Autodesk Inventor part; units mm, degrees
(part 2 of 3)
sketch "Эскиз19" plane through (0, 0, 0) normal (0, 1, 0) x (-1, 0, 0)
  arc A0 (-28.0199, 71.0163) -> (28.0199, 71.0163) centre (0, 104.941) ccw construction
  arc A1 (-23.7825, 76.5969) -> (23.7825, 76.5969) centre (0, 104.941) ccw construction
  line L0 (0, 0) -> (0, 95.3237) construction
  circle A2 centre (0, 56.2966) radius 3.05 construction
  circle A3 centre (0, 56.2966) radius 1.55 construction
  arc A4 (-0.6161, 51.9466) -> (0.6161, 51.9466) centre (0, 53.8493) ccw construction
  arc A5 (-0.6161, 59.3045) -> (0.6161, 59.3045) centre (0, 61.2072) ccw construction
  line L1 (0, 59.2072) -> (0, 51.8493) construction
  arc A6 (0.6251, 60.6437) -> (-0.6251, 60.6437) centre (0, 58.7439) ccw construction
  line L2 (0, 60.7439) -> (0, 51.8493) construction
  line L3 (0, 56.2966) -> (1.525, 58.938) construction
  line L4 (0, 56.2966) -> (-1.525, 58.938) construction
  line L5 (0, 56.2966) -> (-3.05, 56.2966) construction
  line L6 (0, 56.2966) -> (-1.525, 53.6552) construction
  line L7 (0, 56.2966) -> (1.525, 53.6552) construction
  line L8 (0, 56.2966) -> (3.05, 56.2966) construction
  line L9 (1.525, 58.938) -> (3.05, 56.2966) construction
  line L10 (1.525, 53.6552) -> (3.05, 56.2966) construction
  line L11 (1.525, 53.6552) -> (-1.525, 53.6552) construction
  line L12 (-1.525, 53.6552) -> (-3.05, 56.2966) construction
  line L13 (-3.05, 56.2966) -> (-1.525, 58.938) construction
  line L14 (-1.525, 58.938) -> (1.525, 58.938) construction
  arc A7 (0, 51.2466) -> (4.3734, 53.7716) centre (0, 56.2966) ccw construction
  arc A8 (-28.0199, 71.0163) -> (28.0199, 71.0163) centre (0, 104.941) ccw construction
  line L15 (9.0567, 61.8832) -> (4.3734, 53.7716) construction
  line L16 (-9.0567, 61.8832) -> (-4.3734, 53.7716) construction
  arc A9 (-4.3734, 53.7716) -> (0, 51.2466) centre (0, 56.2966) ccw construction
  arc A10 (4.3734, 53.7716) -> (-4.3734, 53.7716) centre (0, 56.2966) ccw construction
  arc A11 (-9.0567, 61.8832) -> (9.0567, 61.8832) centre (0, 104.941) ccw construction
  arc A12 (-9.0567, 61.8832) -> (9.0567, 61.8832) centre (0, 104.941) ccw construction
  line L17 (0, 57.8466) -> (0, 54.7466) construction
  circle A13 centre (-20.558, 60.8542) radius 3.25 construction
  circle A14 centre (-20.558, 60.8542) radius 1.7
  line L18 (-19.3274, 63.4932) -> (-22.4408, 56.8165) construction
  line L19 (-18.6752, 64.8919) -> (-22.4408, 56.8165) construction
  line L20 (-20.558, 60.8542) -> (-17.8958, 62.7183) construction
  line L21 (-20.558, 60.8542) -> (-20.8413, 64.0918) construction
  line L22 (-20.558, 60.8542) -> (-23.5035, 62.2277) construction
  line L23 (-20.558, 60.8542) -> (-23.2203, 58.9901) construction
  line L24 (-20.558, 60.8542) -> (-20.2748, 57.6166) construction
  line L25 (-20.558, 60.8542) -> (-17.6125, 59.4807) construction
  line L26 (-17.8958, 62.7183) -> (-17.6125, 59.4807)
  line L27 (-20.2748, 57.6166) -> (-17.6125, 59.4807)
  line L28 (-20.2748, 57.6166) -> (-23.2203, 58.9901)
  line L29 (-23.2203, 58.9901) -> (-23.5035, 62.2277)
  line L30 (-23.5035, 62.2277) -> (-20.8413, 64.0918)
  line L31 (-20.8413, 64.0918) -> (-17.8958, 62.7183)
  arc A15 (-22.7768, 56.0961) -> (-17.5013, 56.5858) centre (-20.558, 60.8542) ccw
  line L32 (-9.8579, 62.0595) -> (-17.5013, 56.5858)
  line L33 (-26.4019, 69.7424) -> (-25.788, 60.3966)
  arc A16 (-25.788, 60.3966) -> (-22.7768, 56.0961) centre (-20.558, 60.8542) ccw
  arc A17 (-17.5013, 56.5858) -> (-25.788, 60.3966) centre (-20.558, 60.8542) ccw construction
  arc A18 (-26.3973, 69.6727) -> (-9.931, 62.0072) centre (0, 104.8583) ccw construction
  arc A19 (-26.3973, 69.6727) -> (-9.931, 62.0072) centre (0, 104.8583) ccw construction
  line L34 (-19.8396, 62.3949) -> (-21.2765, 59.3135) construction
  arc A20 (-26.4052, 69.7449) -> (-9.8579, 62.0595) centre (0, 104.941) ccw
  line L35 (20.558, 60.8542) -> (20.8413, 64.0918) construction
  line L36 (20.8413, 64.0918) -> (17.8958, 62.7183)
  line L37 (23.5035, 62.2277) -> (20.8413, 64.0918)
  line L38 (20.558, 60.8542) -> (23.5035, 62.2277) construction
  circle A21 centre (20.558, 60.8542) radius 1.7
  line L39 (20.558, 60.8542) -> (23.2203, 58.9901) construction
  line L40 (20.2748, 57.6166) -> (23.2203, 58.9901)
  line L41 (19.3274, 63.4932) -> (22.4408, 56.8165) construction
  circle A22 centre (20.558, 60.8542) radius 3.25 construction
  line L42 (18.6752, 64.8919) -> (22.4408, 56.8165) construction
  arc A23 (25.788, 60.3966) -> (17.5013, 56.5858) centre (20.558, 60.8542) ccw construction
  arc A24 (22.7768, 56.0961) -> (25.788, 60.3966) centre (20.558, 60.8542) ccw
  line L43 (20.558, 60.8542) -> (17.8958, 62.7183) construction
  line L44 (26.4019, 69.7424) -> (25.788, 60.3966)
  line L45 (23.2203, 58.9901) -> (23.5035, 62.2277)
  arc A25 (9.931, 62.0072) -> (26.3973, 69.6727) centre (0, 104.8583) ccw construction
  arc A26 (9.931, 62.0072) -> (26.3973, 69.6727) centre (0, 104.8583) ccw construction
  line L46 (19.8396, 62.3949) -> (21.2765, 59.3135) construction
  line L47 (20.558, 60.8542) -> (20.2748, 57.6166) construction
  line L48 (20.558, 60.8542) -> (17.6125, 59.4807) construction
  line L49 (17.8958, 62.7183) -> (17.6125, 59.4807)
  line L50 (20.2748, 57.6166) -> (17.6125, 59.4807)
  line L51 (9.8579, 62.0595) -> (17.5013, 56.5858)
  arc A27 (17.5013, 56.5858) -> (22.7768, 56.0961) centre (20.558, 60.8542) ccw
  arc A28 (9.8579, 62.0595) -> (26.4052, 69.7449) centre (0, 104.941) ccw
  point P0 (0, 55.5283)
  point P1 (-20.8841, 60.1549)
  point P2 (-9.9889, 62.0899)
  point P3 (20.8841, 60.1549)
  point P4 (9.9889, 62.0899)
  point P5 (9.9889, 62.0899)
  point P6 (-9.9889, 62.0899)
  dimension "d154" = 6.1
  dimension "d155" = 3.1
  dimension "d166" = 360
  dimension "d168" = 2
  dimension "d169" = 30
  dimension "d178" = 6.5
  dimension "d179" = 3.4
  dimension "d180" = 360
  dimension "d181" = 2
  constraints: 102 end point, 56 point on circle, 32 symmetric about line, 23 centre point, 15 point on line, 12 coincident, 6 parallel, 4 midpoint, 4 tangent, 2 perpendicular, 1 collinear, 1 vertical, 47 other
  measures "d154" diameter of A2
  measures "d155" diameter of A3
  measures "d168" radial gap between concentric circles of A7 A2
  measures "d169" angle of L0 L15
  measures "d178" diameter of A13
  measures "d179" diameter of A14
  measures "d181" radial gap between concentric circles of A15 A13
extrude "Выдавливание15" add sketch "Эскиз19" along normal blind 3 contours L26 L27 L28 L29 L30 L31 | L37 L45 L40 L50 L49 L36
extrude "Выдавливание16" add sketch "Эскиз19" along normal blind 10 contours A16 L33 A20 L32 A15 | A27 L51 A28 L44 A24
ref_plane "РабПлоскость7" through (21.7475, 10, 58.3033) normal (0.9063078, 0, 0.4226183) x (0, 1, 0)
sketch "Эскиз22" plane through (21.7475, 10, 58.3033) normal (0.9063078, 0, 0.4226183) x (0, 1, 0)
  line L0 (-10, 51.459) -> (30.2664, 51.459)
  line L1 (-10, -2.4354) -> (-10, 0.1896) construction
  line L2 (-10, -2.4354) -> (-5, -2.4354) construction
  line L3 (-10, -2.4354) -> (0, -2.4354) construction
  line L4 (-5, -2.4354) -> (9.5622, -2.4354) construction
  line L5 (0, 7.459) -> (0, 8.4003) construction
  line L6 (-5, -2.4354) -> (5, -2.4354)
  line L7 (-5, -2.4354) -> (0, 7.459)
  line L8 (0, 7.459) -> (20, 7.459) construction
  line L9 (0, 7.459) -> (5, 7.459)
  line L10 (5, 7.459) -> (5, -2.4354)
  point P0 (-10, -43.6499)
  dimension "d190" = 5
  dimension "d191" = 10
  constraints: 14 end point, 3 point on line, 1 horizontal, 1 midpoint, 1 perpendicular
  measures "d190" distance of L1.start L2.end
  measures "d191" distance of L2.end L6.end
ref_plane "РабПлоскость9" through (-21.7475, 10, 58.3033) normal (-0.9063078, 0, 0.4226183) x (0, -1, 0)
sketch "Эскиз25" plane through (-21.7475, 10, 58.3033) normal (-0.9063078, 0, 0.4226183) x (0, -1, 0)
  line L0 (0, 7.459) -> (-20, 7.459) construction
  line L1 (10, -2.4354) -> (0, -2.4354) construction
  line L2 (10, 0.2379) -> (10, -2.4354) construction
  line L3 (10, -2.4354) -> (5, -2.4354) construction
  line L4 (0, 8.4291) -> (0, 7.459) projected
  line L5 (5, -2.4354) -> (0, 7.459)
  line L6 (0, 7.459) -> (-5, 7.459)
  line L7 (10, 51.459) -> (0, 51.459)
  line L8 (10, 0.2379) -> (10, 0.1896) projected
  line L9 (10, 0.1896) -> (0, 0.1896) projected
  line L10 (0, 0.2379) -> (0, 0.1896) projected
  line L11 (10, 0.2379) -> (0, 0.2379) projected
  line L12 (10, -2.4354) -> (0, -2.4354) projected
  line L13 (5, -2.4354) -> (-4.0389, -6.1705)
  line L14 (-4.0389, -6.1705) -> (-5, 7.459)
  point P0 (10, -43.6499)
  dimension "d192" = 5
  dimension "d193" = 5
  dimension "d194" = 10
  constraints: 12 end point, 1 horizontal, 1 midpoint, 1 point on line
  measures "d192" distance of L1.start L3.end
  measures "d193" distance of L0.start L6.end
  measures "d194" distance of L7.start L7.end
ref_plane "РабПлоскость10" through (0, 0, 69.1191) normal (1, 0, 0) x (0, -1, 0)
sketch "Эскиз26" plane through (0, 0, 69.1191) normal (1, 0, 0) x (0, -1, 0)
  line L0 (0, 8.178) -> (-30, 8.178) projected
  line L1 (0, 17.8725) -> (0, 15.3475) construction
  line L2 (0, 17.8725) -> (0, 15.3475) construction
  line L3 (0, 69.1191) -> (0, -26.2046) construction
  line L4 (0, 8.178) -> (0, 7.0595) projected
  line L5 (0, 8.178) -> (0, 17.8725)
  line L6 (0, 17.8725) -> (-5, 17.8725) construction
  line L7 (0, 17.8725) -> (5, 17.8725) construction
  line L8 (0, 8.178) -> (-10, 8.178)
  line L9 (-10, 8.178) -> (-15, 8.178)
  line L10 (-10, 8.178) -> (-5, 17.8725)
  line L11 (-5, 17.8725) -> (-15, 27.2299)
  line L12 (-15, 27.2299) -> (-15, 8.178)
  line L13 (-18, 0.4099) -> (-28, 0.4099) projected
  line L14 (-28, 0.4099) -> (-28, 0.4099) projected
  line L15 (-28, 0.4099) -> (-18, 0.4099) projected
  line L16 (-18, 0.4099) -> (-18, 0.4099) projected
  line L17 (0, -7.4778) -> (0, -7.4778) projected
  line L18 (0, -7.4778) -> (-30, -7.4778) projected
  line L19 (-30, -7.4778) -> (-30, -7.4778) projected
  line L20 (0, -7.4778) -> (-30, -7.4778) projected
  line L21 (0, -35.822) -> (-10, -35.822) projected
  line L22 (0, -35.822) -> (-10, -35.822)
  dimension "d195" = 5
  dimension "d196" = 180
  dimension "d197" = 10
  dimension "d198" = 5
  constraints: 18 end point, 3 collinear, 1 horizontal, 1 midpoint, 1 perpendicular, 1 point on line
  measures "d195" distance of L1.start L6.end
  measures "d196" angle of L6 L7
  measures "d197" distance of L0.start L8.end
  measures "d198" distance of L8.end L9.end
revolve "Вращение2" cut sketch "Эскиз26" angle 80 mid plane about axis through (0, 0, 104.941) along (0, 1, 0)
sketch "Эскиз29" plane through (76.014, 0, 44.1942) normal (0.7071068, 0, 0.7071068) x (0.7071068, 0, -0.7071068)
  circle A0 centre (-22.5, 11.2) radius 3.75 projected
  circle A1 centre (-22.5, 11.2) radius 25 construction
  point P0 (-22.5, 0)
  dimension "d240" = 50
  constraints: 1 centre point, 1 coincident
  measures "d240" diameter of A1
sketch "Эскиз30" plane through (0, 0, 0) normal (0, 1, 0) x (-1, 0, 0)
  line L0 (-34.2947, -83.085) -> (-38.3657, -87.156) projected
  arc A0 (-34.2947, -83.085) -> (-34.2947, -76.014) centre (-37.8302, -79.5495) ccw projected
  line L1 (-34.2947, -76.014) -> (-76.014, -34.2947) projected
  arc A1 (-76.014, -34.2947) -> (-83.085, -34.2947) centre (-79.5495, -37.8302) ccw projected
  line L2 (-83.085, -34.2947) -> (-87.156, -38.3657) projected
  spline S0 degree 2 poles (-87.5645, -48.6736) (-91.1, -52.2091) (-92.5543, -49.5852) knots 1 1 1 2 2 2 projected
  line L3 (-85.2064, -46.3155) -> (-87.5645, -48.6736) projected
  arc A2 (-73.8927, -46.3155) -> (-85.2064, -46.3155) centre (-79.5495, -51.9723) ccw projected
  line L4 (-46.3155, -73.8927) -> (-73.8927, -46.3155) projected
  arc A3 (-46.3155, -85.2064) -> (-46.3155, -73.8927) centre (-51.9723, -79.5495) ccw projected
  spline S1 degree 2 poles (-48.6736, -87.5645) (-52.2091, -91.1) (-48.7014, -93.0224) knots 1 1 1 2 2 2 projected
  line L5 (-48.6736, -87.5645) -> (-46.3155, -85.2064) projected
  arc A4 (-92.5543, 49.5852) -> (-92.5543, -49.5852) centre (0, 0) ccw construction
  arc A5 (-48.7014, -93.0224) -> (48.7014, -93.0224) centre (0, 0) ccw construction
  line L6 (-38.3657, -87.156) -> (-45.7288, -94.5192)
  line L7 (-87.156, -38.3657) -> (-94.5192, -45.7288)
  line L8 (-92.5543, -49.5852) -> (-94.5192, -45.7288)
  line L9 (-48.7014, -93.0224) -> (-45.7288, -94.5192)
  line L10 (0, 0) -> (0, 95.3237) construction
  line L11 (34.2947, -83.085) -> (38.3657, -87.156)
  arc A6 (34.2947, -76.014) -> (34.2947, -83.085) centre (37.8302, -79.5495) ccw
  line L12 (34.2947, -76.014) -> (76.014, -34.2947)
  arc A7 (83.085, -34.2947) -> (76.014, -34.2947) centre (79.5495, -37.8302) ccw
  line L13 (83.085, -34.2947) -> (87.156, -38.3657)
  line L14 (85.2064, -46.3155) -> (87.5645, -48.6736)
  arc A8 (85.2064, -46.3155) -> (73.8927, -46.3155) centre (79.5495, -51.9723) ccw
  line L15 (46.3155, -73.8927) -> (73.8927, -46.3155)
  arc A9 (46.3155, -73.8927) -> (46.3155, -85.2064) centre (51.9723, -79.5495) ccw
  line L16 (48.6736, -87.5645) -> (46.3155, -85.2064)
  arc A10 (92.5543, -49.5852) -> (92.5543, 49.5852) centre (0, 0) ccw construction
  arc A11 (-48.7014, -93.0224) -> (48.7014, -93.0224) centre (0, 0) ccw construction
  line L17 (38.3657, -87.156) -> (45.7288, -94.5192)
  line L18 (87.156, -38.3657) -> (94.5192, -45.7288)
  line L19 (92.5543, -49.5852) -> (94.5192, -45.7288)
  line L20 (48.7014, -93.0224) -> (45.7288, -94.5192)
  spline S2 degree 2 poles (87.5645, -48.6736) (91.1, -52.2091) (92.5543, -49.5852) knots 1 1 1 2 2 2 projected
  spline S3 degree 2 poles (48.6736, -87.5645) (52.2091, -91.1) (48.7014, -93.0224) knots 1 1 1 2 2 2 projected
  constraints: 28 end point, 25 symmetric about line, 18 point on circle, 6 centre point, 2 coincident, 2 collinear, 6 other
extrude "Выдавливание20" add sketch "Эскиз30" along normal blind 30
pattern_circular "Круговой массив3" count 4 over 360 about axis through (0, -10, 0) along (0, 1, 0) of "Выдавливание2", "Выдавливание3", "Выдавливание21"
ref_plane "РабПлоскость11" through (0, 30, 0) normal (0, 1, 0) x (1, 0, 0)
extrude "Выдавливание22" add sketch "bottom_frame" against normal blind 2 contours S1 L4 A7 L5 A1 L1 S0 A4 S7 L2 A3 L33 A15 L32 S6 A18 S2 L20 A17 L21 A11 L24 S3 A12 S5 L17 A10 L27 A5 L3 S4 A6 A44 L40 A45 L39 A21 L37 A20 L36 A19 A0 | L76 L105 L69 L51 L73 A46 L71 A47 L74 L70 L110 L87 L58 L82 A54 L85 A55 L83 L84 L108 L92 L50 L93 A60 L90 A59 L88 L89 L112 L80 L41 L81 A52 L79 A50 L77
sketch "upper_frame" plane through (0, 30, 0) normal (0, 1, 0) x (1, 0, 0)
  line L0 (85.2064, 46.3155) -> (87.5645, 48.6736)
  arc A0 (73.8927, 46.3155) -> (85.2064, 46.3155) centre (79.5495, 51.9723) ccw
  line L1 (46.3155, 73.8927) -> (73.8927, 46.3155)
  line L2 (73.8927, 46.3155) -> (46.3155, 73.8927) construction
  line L3 (48.6736, 87.5645) -> (46.3155, 85.2064)
  line L4 (48.6736, 87.5645) -> (52.2091, 91.1) construction
  spline S0 degree 2 poles (48.6736, 87.5645) (52.2091, 91.1) (48.7014, 93.0224) knots 1 1 1 2 2 2
  line L5 (52.2091, 91.1) -> (48.7014, 93.0224) construction
  line L6 (87.5645, 48.6736) -> (91.1, 52.2091) construction
  spline S1 degree 2 poles (87.5645, 48.6736) (91.1, 52.2091) (92.5543, 49.5852) knots 1 1 1 2 2 2
  line L7 (91.1, 52.2091) -> (92.5543, 49.5852) construction
  arc A1 (92.5543, 49.5852) -> (48.7014, 93.0224) centre (0, 0) ccw construction
  arc A2 (91.2033, 35.8602) -> (35.8602, 91.2033) centre (0, 0) ccw construction
  line L8 (34.2947, 76.014) -> (76.014, 34.2947)
  line L9 (76.014, 34.2947) -> (34.2947, 76.014) construction
  line L10 (19.799, 36.7696) -> (46.669, 63.6396)
  line L11 (42.4264, 67.8823) -> (12.0208, 37.4767)
  arc A3 (-34.6482, -12.0208) -> (-37.4767, -12.0208) centre (-36.0624, -13.435) ccw
  line L12 (-36.0624, 13.435) -> (-36.0624, -13.435) construction
  line L13 (-38.5624, 11.7401) -> (-33.5624, 11.7401) construction
  line L14 (-33.5624, -10.7237) -> (-38.5624, -10.7237) construction
  line L15 (-36.0624, 11.7401) -> (-36.0624, -10.7237) construction
  arc A4 (33.9411, 19.799) -> (36.7696, 19.799) centre (35.3553, 21.2132) ccw
  arc A5 (19.799, 36.7696) -> (19.799, 33.9411) centre (21.2132, 35.3553) ccw
  line L16 (33.9411, 19.799) -> (19.799, 33.9411)
  line L17 (34.6482, 12.0208) -> (12.0208, 34.6482)
  arc A6 (90.4123, 37.7305) -> (87.156, 38.3657) centre (88.5702, 36.9514) ccw
  line L18 (90.4123, 37.7305) -> (91.2033, 35.8602)
  line L19 (83.085, 34.2947) -> (87.156, 38.3657)
  line L20 (36.7696, 19.799) -> (63.6396, 46.669)
  line L21 (37.4767, 12.0208) -> (67.8823, 42.4264)
  line L22 (-36.7696, 19.799) -> (-63.6396, 46.669)
  line L23 (-37.4767, 12.0208) -> (-67.8823, 42.4264)
  line L24 (-42.4264, 67.8823) -> (-12.0208, 37.4767)
  line L25 (0, 0) -> (-60.1041, 60.1041) construction
  line L26 (-19.799, 36.7696) -> (-46.669, 63.6396)
  arc A7 (34.2947, 83.085) -> (34.2947, 76.014) centre (37.8302, 79.5495) ccw
  arc A8 (46.3155, 85.2064) -> (46.3155, 73.8927) centre (51.9723, 79.5495) ccw
  line L27 (46.3155, 85.2064) -> (48.6736, 87.5645) construction
  line L28 (34.2947, 83.085) -> (38.3657, 87.156)
  arc A9 (38.3657, 87.156) -> (37.7305, 90.4123) centre (36.9514, 88.5702) ccw
  line L29 (37.7305, 90.4123) -> (35.8602, 91.2033)
  line L30 (-37.7305, 90.4123) -> (-35.8602, 91.2033)
  arc A10 (48.7014, 93.0224) -> (-48.7014, 93.0224) centre (0, 0) ccw
  arc A11 (35.8602, 91.2033) -> (-35.8602, 91.2033) centre (0, 0) ccw
  arc A12 (-36.7696, 19.799) -> (-33.9411, 19.799) centre (-35.3553, 21.2132) ccw
  arc A13 (-19.799, 33.9411) -> (-19.799, 36.7696) centre (-21.2132, 35.3553) ccw
  arc A14 (-12.0208, 34.6482) -> (-12.0208, 37.4767) centre (-13.435, 36.0624) ccw
  line L31 (-33.9411, 19.799) -> (-19.799, 33.9411)
  line L32 (-34.6482, 12.0208) -> (-12.0208, 34.6482)
  arc A15 (12.0208, 37.4767) -> (12.0208, 34.6482) centre (13.435, 36.0624) ccw
  line L33 (-37.4767, -12.0208) -> (-25.4558, 0) construction
  line L34 (-32.5269, -14.1421) -> (14.1421, 32.5269) construction
  line L35 (-14.1421, 32.5269) -> (32.5269, -14.1421) construction
  line L36 (-12.0208, 37.4767) -> (37.4767, -12.0208) construction
  line L37 (17.477, -64.7643) -> (0.6161, -59.3045)
  arc A16 (0.6161, -59.3045) -> (-0.6161, -59.3045) centre (0, -61.2072) ccw
  line L38 (-17.477, -64.7643) -> (-0.6161, -59.3045)
  arc A17 (12.0208, -34.6482) -> (12.0208, -37.4767) centre (13.435, -36.0624) ccw
  arc A18 (-12.0208, -37.4767) -> (-12.0208, -34.6482) centre (-13.435, -36.0624) ccw
  arc A19 (-48.7014, -93.0224) -> (-45.42, -94.668) centre (0, 0) ccw
  line L39 (0, 0) -> (0, -95.3237) construction
  arc A20 (-91.2033, -35.8602) -> (91.2033, -35.8602) centre (0, 0) ccw construction
  line L40 (-98, 0) -> (98, 0) construction
  line L41 (0, 0) -> (-74.2462, -74.2462) construction
  arc A21 (-73.8927, -46.3155) -> (-85.2064, -46.3155) centre (-79.5495, -51.9723) ccw
  line L42 (-85.2064, -46.3155) -> (-87.5645, -48.6736)
  line L43 (52.2091, -91.1) -> (48.7014, -93.0224) construction
  spline S2 degree 2 poles (48.6736, -87.5645) (52.2091, -91.1) (48.7014, -93.0224) knots 1 1 1 2 2 2
  line L44 (48.6736, -87.5645) -> (52.2091, -91.1) construction
  arc A22 (46.3155, -73.8927) -> (46.3155, -85.2064) centre (51.9723, -79.5495) ccw
  line L45 (48.6736, -87.5645) -> (46.3155, -85.2064)
  arc A23 (45.42, -94.668) -> (48.7014, -93.0224) centre (0, 0) ccw
  line L46 (46.3155, -73.8927) -> (73.8927, -46.3155)
  arc A24 (85.2064, -46.3155) -> (73.8927, -46.3155) centre (79.5495, -51.9723) ccw
  line L47 (85.2064, -46.3155) -> (87.5645, -48.6736)
  spline S3 degree 2 poles (87.5645, -48.6736) (91.1, -52.2091) (92.5543, -49.5852) knots 1 1 1 2 2 2
  line L48 (87.5645, -48.6736) -> (91.1, -52.2091) construction
  line L49 (91.1, -52.2091) -> (92.5543, -49.5852) construction
  arc A25 (-44.0271, -95.3237) -> (-43.577, -95.5303) centre (0, 0) ccw construction
  arc A26 (-46.3155, -85.2064) -> (-46.3155, -73.8927) centre (-51.9723, -79.5495) ccw
  line L50 (-48.6736, -87.5645) -> (-46.3155, -85.2064)
  spline S4 degree 2 poles (-48.6736, -87.5645) (-52.2091, -91.1) (-48.7014, -93.0224) knots 1 1 1 2 2 2
  line L51 (-48.6736, -87.5645) -> (-52.2091, -91.1) construction
  line L52 (-52.2091, -91.1) -> (-48.7014, -93.0224) construction
  line L53 (-52.2091, -91.1) -> (-48.6736, -87.5645) construction
  line L54 (-52.2091, -91.1) -> (-48.6736, -87.5645) construction
  line L55 (-46.3155, -73.8927) -> (-73.8927, -46.3155)
  line L56 (-91.1, -52.2091) -> (-87.5645, -48.6736) construction
  line L57 (-91.1, -52.2091) -> (-92.5543, -49.5852) construction
  spline S5 degree 2 poles (-87.5645, -48.6736) (-91.1, -52.2091) (-92.5543, -49.5852) knots 1 1 1 2 2 2
  line L58 (-87.5645, -48.6736) -> (-91.1, -52.2091) construction
  arc A27 (36.7696, -19.799) -> (33.9411, -19.799) centre (35.3553, -21.2132) ccw
  arc A28 (-33.9411, -19.799) -> (-36.7696, -19.799) centre (-35.3553, -21.2132) ccw
  arc A29 (-37.4767, 12.0208) -> (-34.6482, 12.0208) centre (-36.0624, 13.435) ccw
  arc A30 (37.4767, -12.0208) -> (34.6482, -12.0208) centre (36.0624, -13.435) ccw
  arc A31 (34.6482, 12.0208) -> (37.4767, 12.0208) centre (36.0624, 13.435) ccw
  arc A32 (92.5543, -49.5852) -> (92.5543, 49.5852) centre (0, 0) ccw
  line L59 (34.6482, -12.0208) -> (12.0208, -34.6482)
  arc A33 (76.014, 34.2947) -> (83.085, 34.2947) centre (79.5495, 37.8302) ccw
  arc A34 (91.2033, -35.8602) -> (91.2033, 35.8602) centre (0, 0) ccw
  line L60 (33.9411, -19.799) -> (19.799, -33.9411)
  arc A35 (-85.2064, 46.3155) -> (-73.8927, 46.3155) centre (-79.5495, 51.9723) ccw
  line L61 (-85.2064, 46.3155) -> (-87.5645, 48.6736)
  arc A36 (-92.5543, 49.5852) -> (-92.5543, -49.5852) centre (0, 0) ccw
  circle A37 centre (0, 0) radius 35 construction
  arc A38 (19.799, -33.9411) -> (19.799, -36.7696) centre (21.2132, -35.3553) ccw
  line L62 (-33.9411, -19.799) -> (-19.799, -33.9411)
  line L63 (-12.0208, -37.4767) -> (37.4767, 12.0208) construction
  line L64 (-14.1421, -32.5269) -> (32.5269, 14.1421) construction
  line L65 (-32.5269, 14.1421) -> (-25.0705, 6.6857) construction
  line L66 (-37.4767, 12.0208) -> (12.0208, -37.4767) construction
  line L67 (-34.6482, -12.0208) -> (-12.0208, -34.6482)
  arc A39 (-19.799, -36.7696) -> (-19.799, -33.9411) centre (-21.2132, -35.3553) ccw
  line L68 (87.156, -38.3657) -> (83.085, -34.2947)
  arc A40 (87.156, -38.3657) -> (90.4123, -37.7305) centre (88.5702, -36.9514) ccw
  line L69 (90.4123, -37.7305) -> (91.2033, -35.8602)
  arc A41 (22.4142, -59.3148) -> (21.5111, -58.7128) centre (20.8949, -60.6155) ccw
  line L70 (19.799, -36.7696) -> (46.669, -63.6396)
  line L71 (42.4264, -67.8823) -> (12.0208, -37.4767)
  arc A42 (18.3802, -65.3664) -> (17.477, -64.7643) centre (16.8609, -66.6671) ccw
  line L72 (25.4187, -62.8242) -> (34.1909, -73.0707)
  arc A43 (34.1909, -73.0707) -> (37.1244, -73.1843) centre (35.7102, -71.7701) ccw
  line L73 (34.1909, -73.0707) -> (27.0558, -64.7365) construction
  line L74 (-21.5111, -58.7128) -> (-14.5119, -56.4463) construction
  arc A44 (0.6161, -51.9466) -> (-0.6161, -51.9466) centre (0, -53.8493) ccw
  line L75 (14.5119, -56.4463) -> (0.6161, -51.9466)
  line L76 (-91.1, -52.2091) -> (-92.5543, -49.5852) construction
  line L77 (76.014, -34.2947) -> (37.1244, -73.1843)
  line L78 (36.7696, -19.799) -> (63.6396, -46.669)
  line L79 (37.4767, -12.0208) -> (67.8823, -42.4264)
  arc A45 (-17.477, -64.7643) -> (-18.3802, -65.3664) centre (-16.8609, -66.6671) ccw
  arc A46 (-21.5111, -58.7128) -> (-22.4142, -59.3148) centre (-20.8949, -60.6155) ccw
  line L80 (-22.4142, -59.3148) -> (-25.4187, -62.8242) construction
  line L81 (-42.4264, -67.8823) -> (-12.0208, -37.4767)
  arc A47 (-37.1244, -73.1843) -> (-34.1909, -73.0707) centre (-35.7102, -71.7701) ccw
  line L82 (-36.7696, -19.799) -> (-63.6396, -46.669)
  line L83 (-37.4767, -12.0208) -> (-67.8823, -42.4264)
  line L84 (-76.014, -34.2947) -> (-37.1244, -73.1843)
  line L85 (-19.799, -36.7696) -> (-46.669, -63.6396)
  line L86 (-43.0355, -94.1655) -> (-18.3802, -65.3664)
  arc A48 (-45.42, -94.668) -> (-43.0355, -94.1655) centre (-44.5548, -92.8648) ccw
  line L87 (43.0355, -94.1655) -> (18.3802, -65.3664)
  arc A49 (43.0355, -94.1655) -> (45.42, -94.668) centre (44.5548, -92.8648) ccw
  arc A50 (48.7014, -93.0224) -> (92.5543, -49.5852) centre (0, 0) ccw construction
  line L88 (-52.2091, -91.1) -> (-48.7014, -93.0224) construction
  line L89 (-87.5645, -48.6736) -> (-91.1, -52.2091) construction
  arc A51 (-92.5543, -49.5852) -> (-48.7014, -93.0224) centre (0, 0) ccw construction
  line L90 (-91.1, -52.2091) -> (-52.2091, -91.1) construction
  line L91 (-87.156, -38.3657) -> (-83.085, -34.2947)
  arc A52 (-90.4123, -37.7305) -> (-87.156, -38.3657) centre (-88.5702, -36.9514) ccw
  line L92 (-90.4123, -37.7305) -> (-91.2033, -35.8602)
  arc A53 (-85.9577, 47.0668) -> (-91.2033, 35.8602) centre (0, 0) ccw construction
  line L93 (-87.156, 38.3657) -> (-83.085, 34.2947)
  line L94 (-90.4123, 37.7305) -> (-91.2033, 35.8602)
  arc A54 (-87.156, 38.3657) -> (-90.4123, 37.7305) centre (-88.5702, 36.9514) ccw
  arc A55 (-91.2033, 35.8602) -> (-91.2033, -35.8602) centre (0, 0) ccw
  arc A56 (-83.085, 34.2947) -> (-76.014, 34.2947) centre (-79.5495, 37.8302) ccw
  arc A57 (-34.2947, 76.014) -> (-34.2947, 83.085) centre (-37.8302, 79.5495) ccw
  line L95 (-38.3657, 87.156) -> (-34.2947, 83.085)
  spline S6 degree 2 poles (-48.6736, 87.5645) (-52.2091, 91.1) (-48.7014, 93.0224) knots 1 1 1 2 2 2
  line L96 (-48.6736, 87.5645) -> (-52.2091, 91.1) construction
  line L97 (-52.2091, 91.1) -> (-48.7014, 93.0224) construction
  arc A58 (-37.7305, 90.4123) -> (-38.3657, 87.156) centre (-36.9514, 88.5702) ccw
  line L98 (-48.6736, 87.5645) -> (-46.3155, 85.2064)
  line L99 (-48.6736, 87.5645) -> (-46.3155, 85.2064) construction
  arc A59 (-46.3155, 73.8927) -> (-46.3155, 85.2064) centre (-51.9723, 79.5495) ccw
  line L100 (-76.014, 34.2947) -> (-34.2947, 76.014)
  line L101 (-46.3155, 73.8927) -> (-73.8927, 46.3155)
  line L102 (-46.3155, 73.8927) -> (-73.8927, 46.3155) construction
  line L103 (-73.8927, 46.3155) -> (-46.3155, 73.8927) construction
  arc A60 (-35.8602, 91.2033) -> (-85.9577, 47.0668) centre (0, 0) ccw construction
  line L104 (-87.5645, 48.6736) -> (-91.1, 52.2091) construction
  spline S7 degree 2 poles (-87.5645, 48.6736) (-91.1, 52.2091) (-92.5543, 49.5852) knots 1 1 1 2 2 2
  line L105 (-91.1, 52.2091) -> (-92.5543, 49.5852) construction
  arc A61 (-48.7014, 93.0224) -> (-92.5543, 49.5852) centre (0, 0) ccw construction
  line L106 (0, -51.8493) -> (0, -56.3493) construction
  line L107 (2.0518, -60.1742) -> (0.6251, -60.6437)
  line L108 (-0.6251, -60.6437) -> (-2.0518, -60.1742)
  line L109 (-2.672, -59.9702) -> (-4.5, -60.5621) construction
  line L110 (2.672, -59.9702) -> (4.5, -60.5621) construction
  arc A62 (-0.6251, -60.6437) -> (0.6251, -60.6437) centre (0, -58.7439) ccw
  arc A63 (-2.0518, -60.1742) -> (-3.2931, -60.1713) centre (-2.6769, -62.074) ccw
  arc A64 (3.2931, -60.1713) -> (2.0518, -60.1742) centre (2.6769, -62.074) ccw
  arc A65 (-2.672, -59.9702) -> (-2.5156, -60.0805) centre (0, -56.3493) ccw construction
  arc A66 (2.5156, -60.0805) -> (2.672, -59.9702) centre (0, -56.3493) ccw construction
  arc A67 (0, -51.8493) -> (-0.3604, -51.8638) centre (0, -56.3493) ccw construction
  arc A68 (-1.5976, -52.1425) -> (-2.3373, -52.504) centre (0, -56.3493) ccw construction
  arc A69 (-76.014, -34.2947) -> (-83.085, -34.2947) centre (-79.5495, -37.8302) ccw
  arc A70 (83.085, -34.2947) -> (76.014, -34.2947) centre (79.5495, -37.8302) ccw
  line L111 (0, -105) -> (0, -104.941) construction
  line L112 (0, -104.941) -> (23.6028, -54.3247) construction
  line L113 (0, -104.941) -> (20.5578, -60.8546) construction
  circle A71 centre (20.5578, -60.8546) radius 1.55
  line L114 (20.5578, -60.8546) -> (22.0043, -58.9513) construction
  line L115 (20.5578, -60.8546) -> (14.3139, -69.0704) construction
  line L116 (15.1585, -56.5907) -> (21.0049, -57.3328)
  line L117 (24.842, -61.8893) -> (23.8313, -59.4808)
  arc A72 (24.842, -61.8893) -> (25.4187, -62.8242) centre (28.1154, -60.5155) ccw
  arc A73 (14.5119, -56.4463) -> (15.1585, -56.5907) centre (15.6055, -53.069) ccw
  arc A74 (23.8313, -59.4808) -> (21.0049, -57.3328) centre (20.5578, -60.8546) ccw
  arc A75 (-15.1585, -56.5907) -> (-14.5119, -56.4463) centre (-15.6055, -53.069) ccw
  line L118 (-15.1585, -56.5907) -> (-21.0049, -57.3328)
  arc A76 (-21.0049, -57.3328) -> (-23.8313, -59.4808) centre (-20.5578, -60.8546) ccw
  line L119 (-24.842, -61.8893) -> (-23.8313, -59.4808)
  arc A77 (-25.4187, -62.8242) -> (-24.842, -61.8893) centre (-28.1154, -60.5155) ccw
  line L120 (-25.4187, -62.8242) -> (-34.1909, -73.0707)
  line L121 (-14.5119, -56.4463) -> (-0.6161, -51.9466)
  circle A78 centre (-20.5578, -60.8546) radius 1.55
  circle A79 centre (0, 0) radius 18
  arc A80 (-22.6088, 4.224) -> (-21.6129, -7.8665) centre (0, 0) ccw construction
  line L122 (-37.4767, -12.0208) -> (-26.8701, -1.4142)
  line L123 (-37.4767, 12.0208) -> (-26.8701, 1.4142)
  line L124 (-32.5269, -14.1421) -> (-25.0705, -6.6857)
  line L125 (-32.5269, 14.1421) -> (-25.0705, 6.6857)
  line L126 (-25.4558, 0) -> (-22.8522, -2.6037) construction
  line L127 (-25.4558, 0) -> (-22.8522, 2.6037) construction
  line L128 (-22.8522, 2.6037) -> (12.0208, 37.4767) construction
  line L129 (-25.4558, 0) -> (-22.8522, 2.6037) construction
  line L130 (-21.7769, 7.4159) -> (-21.6129, 7.8665)
  line L131 (-21.7769, -7.4159) -> (-21.6129, -7.8665)
  arc A81 (-21.7769, -7.4159) -> (-25.0705, -6.6857) centre (-23.6563, -8.1) ccw
  arc A82 (-25.0705, 6.6857) -> (-21.7769, 7.4159) centre (-23.6563, 8.1) ccw
  arc A83 (-26.8701, -1.4142) -> (-26.8701, 1.4142) centre (-28.2843, 0) ccw
  line L132 (-25.0705, 6.6857) -> (-18.3848, 0) construction
  arc A84 (-21.6129, 7.8665) -> (-22.6088, 4.224) centre (0, 0) ccw construction
  arc A85 (-21.6129, -7.8665) -> (-7.8665, -21.6129) centre (0, 0) ccw
  line L133 (-21.9203, 3.5355) -> (-21.9203, -3.5355) construction
  circle A86 centre (-21.9203, 0) radius 1.5
  line L134 (12.0208, 37.4767) -> (1.4142, 26.8701)
  line L135 (-12.0208, 37.4767) -> (-1.4142, 26.8701)
  line L136 (14.1421, 32.5269) -> (6.6857, 25.0705)
  line L137 (-14.1421, 32.5269) -> (-6.6857, 25.0705)
  arc A87 (6.6857, 25.0705) -> (7.4159, 21.7769) centre (8.1, 23.6563) ccw
  arc A88 (-7.4159, 21.7769) -> (-6.6857, 25.0705) centre (-8.1, 23.6563) ccw
  arc A89 (-1.4142, 26.8701) -> (1.4142, 26.8701) centre (0, 28.2843) ccw
  line L138 (-12.0208, -37.4767) -> (-1.4142, -26.8701)
  line L139 (12.0208, -37.4767) -> (1.4142, -26.8701)
  line L140 (-14.1421, -32.5269) -> (-6.6857, -25.0705)
  line L141 (14.1421, -32.5269) -> (6.6857, -25.0705)
  arc A90 (-6.6857, -25.0705) -> (-7.4159, -21.7769) centre (-8.1, -23.6563) ccw
  arc A91 (7.4159, -21.7769) -> (6.6857, -25.0705) centre (8.1, -23.6563) ccw
  line L142 (32.5269, -14.1421) -> (25.0705, -6.6857)
  arc A92 (25.0705, -6.6857) -> (21.7769, -7.4159) centre (23.6563, -8.1) ccw
  line L143 (37.4767, -12.0208) -> (26.8701, -1.4142)
  arc A93 (26.8701, 1.4142) -> (26.8701, -1.4142) centre (28.2843, 0) ccw
  line L144 (37.4767, 12.0208) -> (26.8701, 1.4142)
  line L145 (32.5269, 14.1421) -> (25.0705, 6.6857)
  arc A94 (21.7769, 7.4159) -> (25.0705, 6.6857) centre (23.6563, 8.1) ccw
  arc A95 (1.4142, -26.8701) -> (-1.4142, -26.8701) centre (0, -28.2843) ccw
  line L146 (-7.4159, 21.7769) -> (-7.8665, 21.6129)
  line L147 (7.4159, 21.7769) -> (7.8665, 21.6129)
  line L148 (7.4159, -21.7769) -> (7.8665, -21.6129)
  line L149 (-7.4159, -21.7769) -> (-7.8665, -21.6129)
  line L150 (21.7769, -7.4159) -> (21.6129, -7.8665)
  line L151 (21.7769, 7.4159) -> (21.6129, 7.8665)
  arc A96 (-7.8665, 21.6129) -> (-21.6129, 7.8665) centre (0, 0) ccw
  arc A97 (7.8665, 21.6129) -> (-7.8665, 21.6129) centre (0, 0) ccw construction
  arc A98 (21.6129, 7.8665) -> (7.8665, 21.6129) centre (0, 0) ccw
  arc A99 (21.6129, -7.8665) -> (21.6129, 7.8665) centre (0, 0) ccw construction
  arc A100 (7.8665, -21.6129) -> (21.6129, -7.8665) centre (0, 0) ccw
  arc A101 (-7.8665, -21.6129) -> (7.8665, -21.6129) centre (0, 0) ccw construction
  circle A102 centre (0, 21.9203) radius 1.5
  circle A103 centre (0, -21.9203) radius 1.5
  circle A104 centre (21.9203, 0) radius 1.5
  point P0 (60.1041, 60.1041)
  point P1 (-40.4652, 89.2556)
  point P2 (89.2556, 40.4652)
  point P3 (40.4652, 89.2556)
  point P4 (0, -59.1049)
  point P5 (0, -59.2072)
  point P6 (-18.0135, -64.938)
  point P7 (0, -51.7471)
  point P8 (0, -66.2072)
  point P9 (-89.2556, -40.4652)
  point P10 (39.283, -89.7822)
  point P11 (-60.1041, -60.1041)
  point P12 (-55.1543, -55.1543)
  point P13 (-40.6586, -79.5495)
  point P14 (-79.5495, -40.6586)
  point P15 (43.577, -95.5303)
  point P16 (80.9637, -32.1734)
  point P17 (78.1353, -32.1734)
  point P18 (55.1543, -55.1543)
  point P19 (-27.0558, -64.7365)
  point P20 (-35.5963, -74.7124)
  point P21 (-78.1353, -32.1734)
  point P22 (-79.5495, -30.7591)
  point P23 (18.0135, -64.938)
  point P24 (44.0271, -95.3237)
  point P25 (-80.9637, -32.1734)
  point P26 (-89.2556, -40.4652)
  point P27 (-89.2556, 40.4652)
  point P28 (60.1041, -60.1041)
  point P29 (-79.5495, -30.7591)
  point P30 (23.0382, -57.5909)
  point P31 (22.7059, -58.0282)
  point P32 (21.4957, -59.6205)
  point P33 (22.8522, -2.6037)
  point P34 (-22.6088, -4.224)
  point P35 (-22.8506, 4.4659)
  point P36 (-22.8506, -4.4659)
  dimension "d322" = 3.1
  dimension "d261" = 16.3348
  dimension "d262" = 27.5
  dimension "d263" = 8
  dimension "d264" = 5
  dimension "d265" = 5
  dimension "d266" = 3
  dimension "d267" = 4
  dimension "d268" = 70
  dimension "d269" = 85
  dimension "d270" = 105
  dimension "d271" = 40
  dimension "d272" = 18.9344
  dimension "d273" = 5.21
  dimension "d274" = 2
  dimension "d275" = 7
  dimension "d276" = 7
  dimension "d277" = 7
  dimension "d278" = 7
  dimension "d279" = 7
  dimension "d280" = 2
  dimension "d281" = 2
  dimension "d282" = 2
  dimension "d283" = 5
  dimension "d284" = 2
  dimension "d285" = 7
  dimension "d286" = 7
  dimension "d287" = 7
  dimension "d288" = 5
  dimension "d289" = 2
  dimension "d290" = 5
  dimension "d291" = 5
  dimension "d292" = 2
  dimension "d293" = 7
  dimension "d294" = 7
  dimension "d295" = 7
  dimension "d296" = 5
  dimension "d297" = 5
  dimension "d298" = 2
  dimension "d299" = 5
  dimension "d300" = 2
  dimension "d301" = 2
  dimension "d302" = 40
  dimension "d303" = 5
  dimension "d304" = 6
  dimension "d305" = 6
  dimension "d306" = 12
  dimension "d307" = 12
  dimension "d308" = 2
  dimension "d309" = 5
  dimension "d310" = 5
  dimension "d311" = 5
  dimension "d312" = 5
  dimension "d313" = 7
  dimension "d315" = 4.5
  dimension "d316" = 2
  dimension "d317" = 5
  dimension "d318" = 5
  dimension "d319" = 0.059
  dimension "d320" = 25
  dimension "d321" = 48.644
  dimension "d323" = 40.567
  dimension "d324" = 1.7087
  dimension "d325" = 120
  dimension "d326" = 3.55
  constraints: 272 end point, 242 point on circle, 115 symmetric about line, 103 centre point, 99 point on line, 84 tangent, 28 parallel, 21 coincident, 12 equal radius, 5 midpoint, 4 collinear, 4 perpendicular, 2 vertical, 1 horizontal, 75 other
  measures "d261" distance of L56.start point (-79.55, -40.659)
  measures "d262" distance of point (-40.659, -79.55) point (-60.104, -60.104)
  measures "d263" radius of A26
  measures "d264" distance of L53.start L50.start
  measures "d265" distance of L56.end L56.start
  measures "d266" distance of L56.start L57.end
  measures "d267" distance of L53.start L52.end
  measures "d268" diameter of A37
  measures "d269" distance of point (-60.104, -60.104) L41.start
  measures "d270" radius of A36
  measures "d271" distance of A25.start point (-18.013, -64.938)
  measures "d272" distance of point (-18.013, -64.938) point (0, -59.105)
  measures "d273" distance of A25.start L52.end
  measures "d274" radius of A48
  measures "d275" radial gap between concentric circles of A36 A20
  measures "d276" distance between parallel lines of L55 L84
  measures "d277" distance between parallel lines of L42 L91
  measures "d278" distance between parallel lines of L80 L86
  measures "d279" distance between parallel lines of L38 L74
  measures "d280" radius of A46
  measures "d281" radius of A44
  measures "d282" radius of A47
  measures "d283" distance of point (-89.256, -40.465) L92.end
  measures "d284" radius of A52
  measures "d285" distance between parallel lines of L93 L61
  measures "d286" distance between parallel lines of L98 L95
  measures "d287" distance between parallel lines of L100 L101
  measures "d288" distance of point (-89.256, 40.465) L94.end
  measures "d289" radius of A54
  measures "d290" radius of A56
  measures "d291" distance of point (-40.465, 89.256) L30.end
  measures "d292" radius of A58
  measures "d293" distance between parallel lines of L1 L8
  measures "d294" distance between parallel lines of L3 L28
  measures "d295" distance between parallel lines of L0 L19
  measures "d296" radius of A7
  measures "d297" distance of point (40.465, 89.256) L29.end
  measures "d298" radius of A9
  measures "d299" distance of point (89.256, 40.465) L18.end
  measures "d300" radius of A6
  measures "d301" radius of A49
  measures "d302" distance between parallel lines of L31 L100
  measures "d303" distance between parallel lines of L31 L32
  measures "d304" distance between parallel lines of L23 L22
  measures "d305" distance between parallel lines of L24 L26
  measures "d306" distance between parallel lines of L25 L26
  measures "d307" distance between parallel lines of L22 L25
  measures "d308" radius of A12
  measures "d309" distance between parallel lines of L36 L35
  measures "d310" distance between parallel lines of L66 L65
  measures "d311" distance between parallel lines of L63 L64
  measures "d312" distance between parallel lines of L33 L34
  measures "d313" distance of point (0, -66.207) point (0, -59.207)
  measures "d315" distance of L106.start L106.end
  measures "d316" radius of A62
  measures "d317" radius of A69
  measures "d318" radius of A70
  measures "d319" distance of L111.start L112.start
  measures "d320" angle of L39 L112
  measures "d321" distance of L112.start L113.end
  measures "d323" angle of L86 L39
  measures "d324" distance of L114.end point (23.038, -57.591)
  measures "d325" angle of L117 L116
  measures "d326" radius of A72